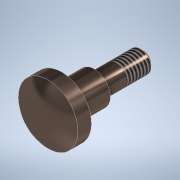
# Autodesk Inventor part: 5輪軸
Saved by Autodesk Inventor 2022 (Build 260153000, 153)
## iProperties
Created: 2023-05-19
Part Number: 5輪軸
Material: 一般
Document SubType Name: Modeling
Designer: USER
Density: 1 g/cm^3
Appearance: 砲銅 - 古董色拋光
Author: USER
Autodesk Inventor part; units mm, degrees
ref_plane "YZ Plane" through (0, 0, 0) normal (1, 0, 0) x (0, 1, 0)
ref_plane "XZ Plane" through (0, 0, 0) normal (0, 1, 0) x (-1, 0, 0)
ref_plane "XY Plane" through (0, 0, 0) normal (0, 0, 1) x (1, 0, 0)
sketch "草圖1" plane through (0, 0, 0) normal (1, 0, 0) x (0, 1, 0)
  line L0 (11, 12.886) -> (0, 12.886)
  line L1 (0, 12.886) -> (0, 7.886)
  line L2 (0, 7.886) -> (11, 7.886)
  line L3 (11, 7.886) -> (11, 12.886)
  line L4 (0, 40.0294) -> (0, 0) construction
  line L5 (84.8092, 0) -> (0, 0) construction
  line L6 (4, -4.114) -> (0, -4.114)
  line L7 (0, -4.114) -> (0, -22.114)
  line L8 (0, -22.114) -> (4, -22.114)
  line L9 (4, -22.114) -> (4, -4.114)
  line L10 (0, 7.886) -> (6, 7.886)
  line L11 (6, 7.886) -> (6, -4.114)
  line L12 (6, -4.114) -> (0, -4.114)
  line L13 (0, -4.114) -> (0, 7.886)
  arc A0 (11, 12.886) -> (0, 16.9425) centre (0, 0) ccw
  line L14 (0, 16.9425) -> (0, -22.114)
  line L15 (0, 16.9425) -> (0, -22.114)
  line L16 (0, 0) -> (14.2081, 0) construction
  point P0 (0, -4.114)
  dimension "d1" = 11
  dimension "d2" = 5
  dimension "d4" = 35
  dimension "d5" = 18
  dimension "d6" = 4
  dimension "d7" = 12
  dimension "d8" = 6
  constraints: 34 end point, 7 equal length, 6 perpendicular, 4 horizontal, 3 collinear, 2 coincident, 2 point on circle, 2 point on line, 1 centre point, 1 vertical
  measures "d1" distance between parallel lines of L1 L3
  measures "d2" distance of L0.start L2.end
  measures "d4" distance between parallel lines of L8 L0
  measures "d5" distance of L6.end L7.end
  measures "d6" distance of L7.end L8.end
  measures "d7" distance of L10.end L11.end
  measures "d8" distance of L11.end L12.end
revolve "迴轉1" add sketch "草圖1" angle 360 about axis through (0, 0, 16.9425) along (0, 0, -1)
chamfer "倒角1" distance 1 angle 45 1 edges at (0, -4, -22.114)
thread "螺紋1" size "M8x1.25" class "6g" standard "ANSI Metric M Profile" length 9 offset 8
